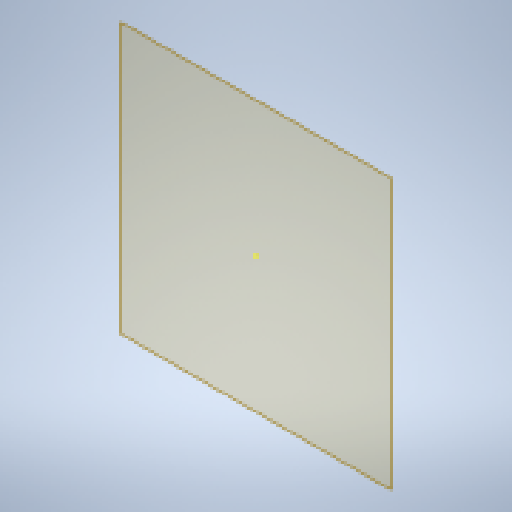
# Autodesk Inventor part: volute_case
Saved by Autodesk Inventor 2023.1 (Build 271208000, 208)
## iProperties
Created: 2024-02-18
Part Number: volute_case
Material: Generic
Document SubType Name: Modeling
Designer: Robot
Density: 1 g/cm^3
Appearance: Default
Author: Robot
Autodesk Inventor part; units mm, degrees
ref_plane "YZ Plane" through (0, 0, 0) normal (1, 0, 0) x (0, 1, 0)
ref_plane "XZ Plane" through (0, 0, 0) normal (0, 1, 0) x (-1, 0, 0)
ref_plane "XY Plane" through (0, 0, 0) normal (0, 0, 1) x (1, 0, 0)
ref_plane "Work Plane1" through (0, 0, 0) normal (0, 0, 1) x (1, 0, 0)
sketch "Sketch1" plane through (0, 0, 0) normal (0, 0, 1) x (1, 0, 0)
  line L0 (0, 0) -> (21, 0)
  line L1 (15.5, 0) -> (15.5, -20)
  circle A0 centre (0, 0) radius 15.5
  line L2 (0, 0) -> (14.0478, -6.5506)
  line L3 (0, 0) -> (0, -16.875)
  line L4 (0, 0) -> (-18.25, 0)
  line L5 (0, 0) -> (0, 19.625)
  arc A1 (-18.25, 0) -> (15.5, 0) centre (-1.375, -0.056) ccw
  arc A2 (21, 0) -> (-18.25, 0) centre (1.375, 0.0482) ccw
  line L6 (21, 0) -> (21, -20)
  line L7 (0, 0) -> (0, -18.875)
  line L8 (0, 0) -> (-20.25, 0)
  line L9 (0, 0) -> (0, 21.625)
  line L10 (0, 0) -> (23, 0)
  line L11 (0, 0) -> (17.5, 0)
  arc A3 (-20.25, 0) -> (17.5, 0) centre (-1.375, -0.0501) ccw
  arc A4 (23, 0) -> (-20.25, 0) centre (1.375, 0.0437) ccw
  line L12 (13.5, -8.0249) -> (13.5, -20)
  line L13 (15.5, -20) -> (13.5, -20)
  line L14 (23, 0) -> (23, -20)
  line L15 (21, -20) -> (23, -20)
  line L16 (21, -20) -> (15.5, -20)
  point P0 (15.5, -8.506)
  point P1 (15.5, -0.112)
  point P2 (21, 0)
  point P3 (13.5, -14.0125)
  point P4 (13.5, -11.6691)
  dimension "d2" = 31
  dimension "d0" = 21
  dimension "d1" = 15.5
  dimension "d3" = 25
  dimension "d4" = 16.875
  dimension "d5" = 18.25
  dimension "d6" = 19.625
  dimension "d7" = 20
  dimension "d8" = 20
  dimension "d9" = 2
  dimension "d10" = 2
  dimension "d11" = 2
  dimension "d12" = 2
  dimension "d13" = 2
  dimension "d16" = 2
  constraints: 34 end point, 13 point on circle, 8 vertical, 4 centre point, 4 horizontal, 4 point on line, 1 coincident, 1 midpoint, 3 other
  measures "d0" distance of L0.start L0.end
  measures "d1" distance of L0.start L1.start
  measures "d3" angle of L0 L2
  measures "d4" distance of L2.start L3.end
  measures "d5" distance of L2.start L4.end
  measures "d6" distance of L2.start L5.end
  measures "d7" distance of L0.end L6.end
  measures "d8" distance of L1.start L1.end
  measures "d9" distance of L7.end L3.end
  measures "d10" distance of L8.end L4.end
  measures "d11" distance of L9.end L5.end
  measures "d12" distance of L10.end L0.end
  measures "d13" distance of L1.start L11.end
  measures "d16" distance from line of L1 point (13.5, -14.012)
extrude "Extrusion1" add sketch "Sketch1" along normal blind 18 contours L1 A3 L12 A1 | L1 L13 L12 A3 | L12 A3 L7 A1 | L7 A3 L8 A1 | L8 A4 L9 A2 | L9 A4 L10 A2 | L10 L14 L15 L6
extrude "Extrusion2" add sketch "Sketch1" along normal blind 3 contours L5 A0 L0 | L0 A0 L2 | L2 A0 L3 | L3 A0 L4 | L4 A0 L5 | A0 L5 A2 L0 | L0 A3 L1 | A1 L3 A0 | L3 A1 L4 A0 | L4 A2 L5 A0 | L0 L6 L16 L1 A3
sketch "Sketch2" plane through (13.5, -20, 0) normal (0, -1, 0) x (1, 0, 0)
  circle A0 centre (4.7788, 10.8992) radius 2.75
  point P0 (-13.5, 0)
  dimension "d19" = 5.5
  constraints: 1 centre point
  measures "d19" diameter of A0
equation "\"d2\" = VoluteCaseInnerSize"
equation "\"d0\" = 0.5 * VoluteCaseOuterSize"
equation "\"d1\" = 0.5 * VoluteCaseInnerSize"
equation "\"d3\" = VoluteStartAngle"
equation "\"d4\" = 0.375 * VoluteCaseInnerSize + 0.125 * VoluteCaseOuterSize"
equation "\"d5\" = 0.25 * VoluteCaseInnerSize + 0.25 * VoluteCaseOuterSize"
equation "\"d6\" = 0.125 * VoluteCaseInnerSize + 0.375 * VoluteCaseOuterSize"
equation "\"d7\" = VoluteOutletLength"
equation "\"d8\" = VoluteOutletLength"
equation "\"d9\" = VoluteWallThickness"
equation "\"d10\" = VoluteWallThickness"
equation "\"d11\" = VoluteWallThickness"
equation "\"d12\" = VoluteWallThickness"
equation "\"d13\" = VoluteWallThickness"
equation "\"d16\" = VoluteWallThickness"
equation "\"d14\" = VoluteBaseWallThickness + VoluteWallDepth"
equation "\"d17\" = VoluteBaseWallThickness"
equation "\"d19\" = OutletRadius"
equation "\"PropHoleDiameter\" = 8.2"
equation "\"PropBladeThickness\" = 1"
equation "\"PropPlateThickness\" = 2"
equation "\"VoluteCaseInnerSize\" = 31"
equation "\"VoluteCaseOuterSize\" = 42"
equation "\"VoluteWallThickness\" = 2"
equation "\"VoluteStartAngle\" = 25deg"
equation "\"VoluteOutletLength\" = 20"
equation "\"VoluteBaseWallThickness\" = 3"
equation "\"VoluteWallDepth\" = 15"
equation "\"OutletRadius\" = 5.5"
body "Solid1"
